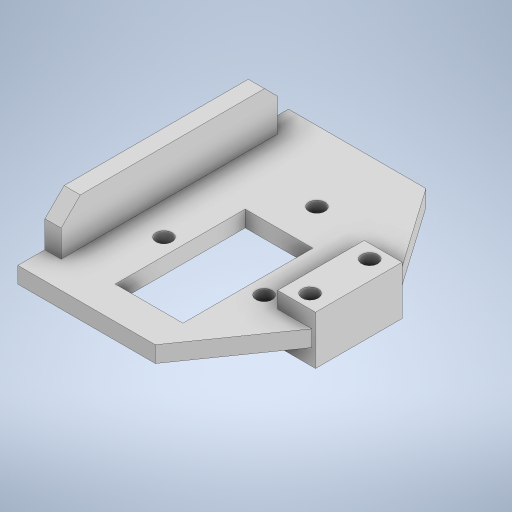
# Autodesk Inventor part: Pinza_pieza1
Saved by Autodesk Inventor 2023 (Build 270158000, 158)
## iProperties
Created: 2024-09-28
Part Number: Pinza_pieza1
Material: Genérico
Document SubType Name: Sheet Metal
Designer: sebas
Density: 1 g/cm^3
Sheet Metal Rule: Por defecto_mm
Appearance: Valor por defecto
Author: sebas
Autodesk Inventor part; units mm, degrees
ref_plane "YZ Plane" through (0, 0, 0) normal (1, 0, 0) x (0, 1, 0)
ref_plane "XZ Plane" through (0, 0, 0) normal (0, 1, 0) x (-1, 0, 0)
ref_plane "XY Plane" through (0, 0, 0) normal (0, 0, 1) x (1, 0, 0)
sketch "Boceto1" plane through (0, 0, 0) normal (1, 0, 0) x (0, 1, 0)
  line L0 (10, 16.4587) -> (10, -17.5667)
  line L1 (10, -17.5667) -> (7.5667, -20)
  line L2 (7.5667, -20) -> (-5.3553, -20)
  line L3 (-5.3553, -20) -> (-10, -15.3553)
  line L4 (-10, -15.3553) -> (-10, 14.7117)
  line L5 (-10, 14.7117) -> (-4.7117, 20)
  line L6 (-4.7117, 20) -> (6.4587, 20)
  line L7 (6.4587, 20) -> (10, 16.4587)
  line L8 (0, 0) -> (31.525, 0) construction
  line L9 (0, 0) -> (0, -54.6434) construction
  dimension "d0" = 135
  dimension "d2" = 135
  dimension "d3" = 135
  dimension "d5" = 40
  dimension "d6" = 20
  constraints: 20 end point, 2 horizontal, 2 parallel, 2 vertical, 1 perpendicular, 2 other
  measures "d0" angle of L0 L7
  measures "d2" angle of L4 L5
  measures "d3" angle of L1 L0
  measures "d5" distance between parallel lines of L2 L6
  measures "d6" distance between parallel lines of L4 L0
extrude "Extrusión1" add sketch "Boceto1" along normal mid plane 3
sketch "Boceto2" plane through (0, 0, 0) normal (0, 1, 0) x (-1, 0, 0)
  line L0 (0, 0) -> (-24, 0) construction
  line L1 (1.5, -25) -> (-23.8963, -25)
  line L2 (-23.8963, -25) -> (-36.5, -7)
  line L3 (-36.5, -7) -> (-36.5, 7)
  line L4 (-36.5, 7) -> (-23.8963, 25)
  line L5 (-23.8963, 25) -> (1.5, 25)
  line L6 (-1.5, 20) -> (1.5, 20) projected
  line L7 (-1.5, -15.3553) -> (-1.5, -20) projected
  line L8 (-1.5, 20) -> (-1.5, -20)
  line L9 (1.5, 20) -> (-1.5, 20)
  line L10 (1.5, -20) -> (1.5, -15.3553) projected
  line L11 (1.5, -20) -> (-1.5, -20) projected
  line L12 (1.5, -20) -> (-1.5, -20)
  line L13 (1.5, -20) -> (1.5, -25)
  line L14 (1.5, 20) -> (1.5, 25)
  line L15 (1.5, 16.4587) -> (1.5, -17.5667) projected
  line L16 (-10.5, 19) -> (-23, 19)
  line L17 (-23, 19) -> (-23, -5)
  line L18 (-23, -5) -> (-10.5, -5)
  line L19 (-10.5, -5) -> (-10.5, 19)
  line L20 (-10.5, 7) -> (-23, 7) construction
  circle A0 centre (-7.5, 7) radius 1.5
  circle A1 centre (-26, 7) radius 1.5
  circle A2 centre (-16.75, -12) radius 1.5
  line L21 (-16.75, -5) -> (-16.75, -34) construction
  dimension "d9" = 50
  dimension "d10" = 38
  dimension "d11" = 145
  dimension "d12" = 145
  dimension "d13" = 12.5
  dimension "d14" = 24
  dimension "d15" = 6
  dimension "d16" = 12
  dimension "d17" = 3
  dimension "d18" = 3
  dimension "d19" = 3
  dimension "d20" = 3
  dimension "d21" = 3
  dimension "d22" = 7
  constraints: 34 end point, 5 equal length, 4 vertical, 3 centre point, 3 midpoint, 2 horizontal, 1 perpendicular, 1 point on line, 1 symmetric about line, 1 other
  measures "d9" distance between parallel lines of L1 L5
  measures "d10" distance between parallel lines of L3 L15
  measures "d11" angle of L2 L3
  measures "d12" angle of L4 L3
  measures "d13" distance between parallel lines of L17 L19
  measures "d14" distance of L18.end L16.start
  measures "d15" distance between parallel lines of L5 L16
  measures "d16" distance between parallel lines of L19 L15
  measures "d17" diameter of A0
  measures "d18" diameter of A1
  measures "d19" distance from line of A0.centre L19
  measures "d20" distance from line of L17 A1.centre
  measures "d21" diameter of A2
  measures "d22" distance from line of L18 A2.centre
extrude "Extrusión2" add sketch "Boceto2" along normal mid plane 3
sketch "Boceto3" plane through (0, 0, 0) normal (0, 1, 0) x (-1, 0, 0)
  line L0 (-36.5, -8) -> (-29.5, -8)
  line L1 (-29.5, -8) -> (-29.5, 8)
  line L2 (-29.5, 8) -> (-36.5, 8)
  line L3 (-36.5, 8) -> (-36.5, -8)
  line L4 (0, 0) -> (-66, 0) construction
  point P0 (-33, -8)
  point P1 (-33, 8)
  dimension "d25" = 7
  dimension "d34" = 8
  dimension "d35" = 8
  constraints: 10 end point, 2 horizontal, 2 midpoint, 2 parallel, 1 perpendicular
  measures "d25" distance of L2.end L1.end
  measures "d34" distance from line of point (-33, -8) L4
  measures "d35" distance from line of point (-33, 8) L4
extrude "Extrusión3" add sketch "Boceto3" along normal mid plane 9
sketch "Boceto4" plane through (0, 4.5, 0) normal (0, 1, 0) x (1, 0, 0)
  circle A0 centre (33, 5.5) radius 1.5
  circle A1 centre (33, -5.5) radius 1.5
  line L0 (-1.5, 15.3553) -> (-1.5, -14.7117) projected
  line L1 (-1.5, 0) -> (97, 0) construction
  line L2 (97, 0) -> (96, 0)
  point P0 (0, 0)
  dimension "d28" = 3
  dimension "d29" = 3
  dimension "d30" = 11
  dimension "d31" = 5.5
  constraints: 4 end point, 2 centre point, 2 point on line, 1 horizontal
  measures "d28" diameter of A0
  measures "d29" diameter of A1
  measures "d30" distance of A1.centre A0.centre
  measures "d31" distance from line of A1.centre L1
extrude "Extrusión4" cut sketch "Boceto4" against normal up to surface (9 mm away)
sketch "Boceto5" plane through (-1.5, 0, 0) normal (-1, 0, 0) x (0, 0, 1)
  circle A0 centre (0, 0) radius 3.5
  dimension "d38" = 7
  constraints: 1 centre point, 1 coincident
  measures "d38" diameter of A0
extrude "Extrusión5" cut sketch "Boceto5" against normal blind 1
equation "\"Radio_pliegue\" = Grosor"
equation "\"Anchura_desahogo_plegado\" = Grosor"
equation "\"Profundidad_desahogo_plegado\" = 0.5 * Grosor"
equation "\"Tamaño_destalonado\" = 4 * Grosor"
equation "\"Remanente_mínimo\" = 2 * Grosor"
equation "\"Radiodetransición\" = Radio_pliegue"
equation "\"Tamaño_de_radio_de_Jacobi\" = Radio_pliegue"
equation "\"TamañoSeparación\" = Grosor"
equation "\"Grosor\" = 0.5"
